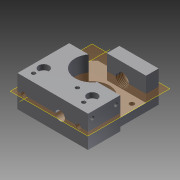
# Autodesk Inventor part: D-036
Saved by Autodesk Inventor 2015 (Build 190159000, 159)
## iProperties
Company: MARCHA TECHNOLOGY
Created: 2014-06-19
Part Number: D-036
Document SubType Name: Modeling
Designer: O.Martin
Density: 1 g/cm^3
Project: WITBOXprinter_K01
Description: CUERPO EXTRUDER
Stock Number: 28655
Mass: 22.3475 g
Surface Area: 90.0971 cm^2
Volume: 22.3475 cm^3
Material: Generic
Appearance: Light Gray
Author: O.Martin
Autodesk Inventor part; units mm, degrees
ref_plane "YZ Plane" through (0, 0, 0) normal (1, 0, 0) x (0, 1, 0)
ref_plane "XZ Plane" through (0, 0, 0) normal (0, 1, 0) x (-1, 0, 0)
ref_plane "XY Plane" through (0, 0, 0) normal (0, 0, 1) x (1, 0, 0)
sketch "Boceto1" plane through (0, 0, 0) normal (0, 0, 1) x (1, 0, 0)
  line L0 (-21.25, 49) -> (21.25, 49)
  line L1 (21.25, 49) -> (21.25, 0)
  line L2 (21.25, 0) -> (-21.25, 0)
  line L3 (-21.25, 0) -> (-21.25, 49)
  circle A0 centre (0, 26.5) radius 11
  line L4 (-15.5, 42) -> (15.5, 42) construction
  line L5 (15.5, 42) -> (15.5, 11) construction
  line L6 (15.5, 11) -> (-15.5, 11) construction
  line L7 (-15.5, 11) -> (-15.5, 42) construction
  circle A1 centre (-15.5, 42) radius 1.75
  circle A2 centre (15.5, 42) radius 1.75
  circle A3 centre (15.5, 11) radius 1.75
  circle A4 centre (-15.5, 11) radius 1.75
  point P0 (0, 0)
  point P1 (0, 0)
  point P2 (0, 42)
  point P3 (-15.5, 26.5)
  dimension "d0" = 42.5
  dimension "d1" = 49
  dimension "d2" = 22
  dimension "d3" = 26.5
  dimension "d4" = 31
  dimension "d5" = 3.5
  constraints: 16 end point, 5 centre point, 5 coincident, 4 parallel, 3 equal radius, 3 midpoint, 3 perpendicular, 2 horizontal, 2 vertical alignment, 1 horizontal alignment
  measures "d0" distance of L1.end L2.end
  measures "d1" distance of L2.end L0.start
  measures "d2" diameter of A0
  measures "d3" distance from line of L2 A0.centre
  measures "d4" distance of L4.start L4.end
  measures "d5" diameter of A1
extrude "Extrusión1" add sketch "Boceto1" along normal blind 20 contours L0 L1 L2 L3 | A1 | A2
sketch "Boceto2" plane through (-21.25, 0, 0) normal (0, -1, 0) x (1, 0, 0)
  line L0 (0, 0) -> (0, 20) projected
  line L1 (42.5, 0) -> (0, 0) projected
  line L2 (3.75, 10) -> (38.75, 10) construction
  line L3 (32.25, 0) -> (10.25, 0) construction
  point P0 (0, 10)
  point P1 (21.25, 10)
  point P2 (21.25, 0)
  dimension "d8" = 35
  constraints: 3 midpoint, 2 coincident, 2 end point, 1 horizontal alignment, 1 parallel, 1 vertical alignment
  measures "d8" distance of L2.start L2.end
hole "Agujero1" at (-17.5, 0, 10) at (17.5, 0, 10) direction (0, 1, 0) diameter 3.242 depth 8 tip angle 118 thread size "M4x0.7" class "6H" standard "ISO Metric profile"
sketch "Boceto3" plane through (0, 0, 20) normal (0, 0, 1) x (1, 0, 0)
  circle A0 centre (0, 26.5) radius 11 projected
  line L0 (21.25, 49) -> (21.25, 0) projected
  line L1 (-21.25, 0) -> (-21.25, 49) projected
  line L2 (-21.25, 39.5) -> (21.25, 39.5)
  line L3 (21.25, 39.5) -> (21.25, 15)
  line L4 (-21.25, 15) -> (-21.25, 39.5)
  line L5 (-21.25, 33) -> (-8.8741, 33)
  line L6 (21.25, 0) -> (-21.25, 0) projected
  line L7 (9.2195, 20.5) -> (21.25, 20.5)
  dimension "d17" = 13
  dimension "d161" = 6
  dimension "d186" = 6.5
  constraints: 10 end point, 4 point on line, 2 parallel, 2 perpendicular, 2 point on circle, 1 horizontal
  measures "d17" distance from line of L2 A0.centre
  measures "d161" distance from line of A0.centre L7
  measures "d186" distance from line of A0.centre L5
extrude "Extrusión2" cut sketch "Boceto3" against normal blind 15 contours A0 L5 L1 L2 L0 L7
sketch "Boceto4" plane through (-21.25, 0, 0) normal (0, -1, 0) x (1, 0, 0)
  line L0 (42.5, 20) -> (0, 20) projected
  line L1 (42.5, 0) -> (0, 0) projected
  line L2 (21.25, 0) -> (21.25, 20) construction
  line L3 (42.5, 0) -> (42.5, 20) projected
  point P0 (27.25, 10)
  point P1 (42.5, 10)
  dimension "d22" = 6
  constraints: 3 midpoint, 2 end point, 1 horizontal alignment
  measures "d22" distance from line of point (27.25, 10) L2
hole "Agujero2" at (6, 0, 10) direction (0, 1, 0) diameter 6 depth 20 tip angle 118
sketch "Boceto5" plane through (-21.25, 49, 20) normal (0, 1, 0) x (1, 0, 0)
  line L0 (0, 20) -> (0, 0) projected
  circle A0 centre (27.25, 10) radius 3 projected
  circle A1 centre (38.75, 10) radius 1.621 projected
  circle A2 centre (3.75, 10) radius 1.621 projected
  line L1 (42.5, 0) -> (0, 0) projected
  line L2 (0, 20) -> (0, 0) projected
  line L3 (42.5, 20) -> (0, 20) projected
  line L4 (42.5, 20) -> (42.5, 0) projected
  point P0 (6.5, 10)
  dimension "d46" = 6.5
  constraints: 1 horizontal alignment
  measures "d46" distance from line of L0 point (6.5, 10)
hole "Agujero3" at (-14.75, 49, 10) direction (0, -1, 0) diameter 5 depth 28.5
sketch "Boceto6" plane through (0, 0, 5) normal (0, 0, 1) x (1, 0, 0)
  line L0 (21.25, 39.5) -> (21.25, 20.5) projected
  arc A0 (9.2195, 20.5) -> (-8.8741, 33) centre (0, 26.5) ccw projected
  point P0 (21.25, 15.5)
  point P1 (17.25, 34.5)
  dimension "d48" = 4
  dimension "d187" = 8
  measures "d48" distance from line of L0 point (17.25, 34.5)
  measures "d187" vertical distance of point (17.25, 34.5) A0.centre
hole "Agujero4" at (17.25, 34.5, 5) direction (0, 0, -1) diameter 3 end through all
sketch "Boceto7" plane through (-21.25, 49, 0) normal (0, 1, 0) x (1, 0, 0)
  line L0 (0, -20) -> (42.5, -20) projected
  line L1 (0, 0) -> (42.5, 0) projected
  line L2 (21.25, 0) -> (21.25, -20) construction
  circle A0 centre (27.25, -10) radius 3 projected
  circle A1 centre (38.75, -10) radius 1.621 projected
  circle A2 centre (3.75, -10) radius 1.621 projected
  line L3 (42.5, -20) -> (0, -20) projected
  line L4 (0, 0) -> (0, -20) projected
  line L5 (42.5, 0) -> (0, 0) projected
  line L6 (42.5, 0) -> (42.5, -20) projected
  constraints: 2 end point, 2 midpoint, 1 coincident
hole "Agujero5" at (6, 49, 10) direction (0, -1, 0) diameter 8.566 depth 15 tip angle 118 thread size "G9.728x0.907" designation "G 1/8" standard "ISO Pipe Threads"
sketch "Boceto15" plane through (0, 0, 20) normal (0, 0, 1) x (1, 0, 0)
  circle A0 centre (-15.5, 11) radius 1.75 projected
  circle A1 centre (15.5, 11) radius 1.75 projected
  line L0 (-21.25, 49) -> (21.25, 49) projected
  line L1 (-21.25, 39.5) -> (21.25, 39.5) projected
  line L2 (21.25, 20.5) -> (21.25, 0) projected
  line L3 (-21.25, 39.5) -> (-21.25, 49) projected
  line L4 (-8.8741, 33) -> (-21.25, 33) projected
  line L5 (-21.25, 0) -> (-21.25, 33) projected
  line L6 (21.25, 0) -> (-21.25, 0) projected
  line L7 (21.25, 20.5) -> (9.2195, 20.5) projected
  arc A2 (-8.8741, 33) -> (9.2195, 20.5) centre (0, 26.5) ccw projected
  line L8 (21.25, 49) -> (21.25, 39.5) projected
  point P0 (15.5, 42)
  constraints: 2 coincident
hole "Agujero10" at (-15.5, 11, 20) at (15.5, 11, 20) direction (0, 0, -1) diameter 3.4 end through all counterbore diameter 6.5 counterbore depth 3.4 clearance for "Tornillo de cabeza hueca DIN EN ISO 4762" size "M3" standard "DIN"
sketch "Boceto16" plane through (0, 0, 20) normal (0, 0, 1) x (1, 0, 0)
  line L0 (21.25, 0) -> (-21.25, 0) projected
  line L1 (21.25, 20.5) -> (21.25, 0) projected
  line L2 (-16, 5) -> (16, 5) construction
  circle A0 centre (15.5, 11) radius 3.25 projected
  point P0 (21.25, 15.5)
  point P1 (-23.75, 0)
  dimension "d130" = 32
  dimension "d131" = 5
  dimension "d139" = 0.5
  constraints: 2 coincident, 2 end point, 1 perpendicular
  measures "d130" distance of L2.start L2.end
  measures "d131" distance between parallel lines of L0 L2
  measures "d139" horizontal distance of point (16, 5) A0.centre
hole "Agujero11" at (-16, 5, 20) at (16, 5, 20) direction (0, 0, -1) diameter 2.459 depth 6 tip angle 118 thread size "M3x0.5" class "6H" standard "ISO Metric profile"
move faces "Desplazar cara3" translate (0, -1.5, 0) faces at (1.6583, 49, 18.0528)
sketch "Boceto19" plane through (0, 0, 20) normal (0, 0, 1) x (1, 0, 0)
  circle A0 centre (15.5, 11) radius 3.25 projected
  line L0 (10.283, 39.5) -> (1.717, 39.5) projected
  point P0 (6, 11)
  point P1 (6, 39.5)
  constraints: 1 horizontal alignment, 1 midpoint, 1 vertical alignment
hole "Agujero13" at (6, 11, 20) direction (0, 0, -1) diameter 2.459 depth 8 tip angle 118 thread size "M3x0.5" class "6H" standard "ISO Metric profile"
sketch "Boceto20" plane through (0, 0, 20) normal (0, 0, 1) x (1, 0, 0)
  line L0 (-21.25, 39.5) -> (21.25, 39.5) projected
  line L1 (21.25, 47.5) -> (21.25, 39.5) projected
  line L2 (-21.25, 47.5) -> (21.25, 47.5) projected
  line L3 (-21.25, 39.5) -> (-21.25, 47.5) projected
  line L4 (-3.75, 47.5) -> (-3.75, 39.5)
  dimension "d162" = 25
  constraints: 2 end point, 2 point on line, 1 parallel
  measures "d162" distance between parallel lines of L1 L4
extrude "Extrusión9" cut sketch "Boceto20" against normal up to surface (15 mm away) contours L3 L2 L4 L0
sketch "Boceto21" plane through (21.25, 0, 20) normal (1, 0, 0) x (0, 0, -1)
  line L0 (15, 20.5) -> (0, 20.5) projected
  line L1 (0, 20.5) -> (0, 0) projected
  line L2 (20, 0) -> (0, 0) projected
  line L3 (20, 47.5) -> (20, 0) projected
  line L4 (15, 20.5) -> (20, 20.5)
  constraints: 2 end point, 1 perpendicular, 1 point on line
extrude "Extrusión10" add sketch "Boceto21" along normal blind 2.5
chamfer "Chaflán4" distance 4 angle 45 1 edges at (-21.25, 47.5, 2.5)
sketch "Boceto22" plane through (23.75, 0, 20) normal (1, 0, 0) x (0, 0, -1)
  line L0 (0, 0) -> (0, 20.5) projected
  line L1 (4, 2.75) -> (4, 17.75) construction
  line L2 (0, 0) -> (0, 33) construction
  point P0 (4, 10.25)
  point P1 (0, 10.25)
  dimension "d173" = 4
  dimension "d174" = 15
  constraints: 2 coincident, 2 end point, 2 midpoint, 1 horizontal alignment, 1 parallel
  measures "d173" distance between parallel lines of L2 L1
  measures "d174" distance of L1.start L1.end
hole "Agujero14" at (23.75, 17.75, 16) at (23.75, 2.75, 16) direction (-1, 0, 0) diameter 2.459 depth 6 tip angle 118 thread size "M3x0.5" class "6H" standard "ISO Metric profile"
ref_plane "Plano de trabajo2" through (0, 0, 10) normal (0, 0, 1) x (1, 0, 0)
hole "Agujero15" at (6, 47.5, 10) direction (0, -1, 0) diameter 10 depth 3
sketch "Boceto25" plane through (-21.25, 0, 0) normal (-1, 0, 0) x (0, 0, 1)
  line L0 (0, 0) -> (0, 43.5) projected
  line L1 (0, 0) -> (20, 0) projected
  point P0 (6, 26.5)
  dimension "d202" = 26.5
  dimension "d203" = 6
  measures "d202" distance from line of point (6, 26.5) L1
  measures "d203" distance from line of L0 point (6, 26.5)
hole "Agujero16" at (-21.25, 26.5, 6) direction (1, 0, 0) diameter 3 depth 12 tip angle 118
body "Solid1"
